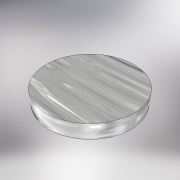
# Autodesk Inventor part: Magnet_10mm
Saved by Autodesk Inventor 2022.1 (Build 261234020, 234B)
## iProperties
Created: 2022-04-27
Part Number: Magnet_10mm
Material: Stainless Steel
Document SubType Name: Modeling
Designer: Remo
Density: 8 g/cm^3
Appearance: Polished Brushed
Author: Remo
Autodesk Inventor part; units mm, degrees
ref_plane "YZ Plane" through (0, 0, 0) normal (1, 0, 0) x (0, 1, 0)
ref_plane "XZ Plane" through (0, 0, 0) normal (0, 1, 0) x (-1, 0, 0)
ref_plane "XY Plane" through (0, 0, 0) normal (0, 0, 1) x (1, 0, 0)
sketch "Sketch1" plane through (0, 0, 0) normal (0, 1, 0) x (-1, 0, 0)
  circle A0 centre (0, 0) radius 5
  dimension "d0" = 10
  constraints: 1 centre point, 1 coincident
  measures "d0" diameter of A0
extrude "Extrusion1" add sketch "Sketch1" along normal blind 1.5
body "Solid1"
